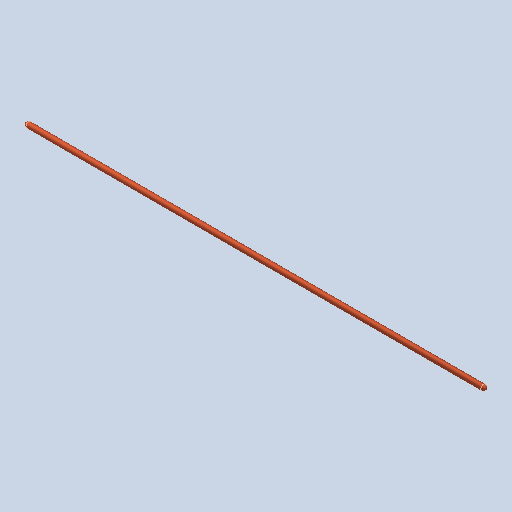
# Autodesk Inventor part: Heat Pipe 250 mm
Saved by Autodesk Inventor 2026.2 (Build 302298010, 298A)
## iProperties
Created: 2026-04-26
Part Number: Heat Pipe 250 mm
Material: Copper, Alloy
Document SubType Name: Modeling
Designer: piete
Density: 8.92 g/cm^3
Appearance: Copper - Satin
Author: piete
Autodesk Inventor part; units mm, degrees
ref_plane "YZ Plane" through (0, 0, 0) normal (1, 0, 0) x (0, 1, 0)
ref_plane "XZ Plane" through (0, 0, 0) normal (0, 1, 0) x (-1, 0, 0)
ref_plane "XY Plane" through (0, 0, 0) normal (0, 0, 1) x (1, 0, 0)
sketch "Sketch1" plane through (0, 0, 0) normal (1, 0, 0) x (0, 1, 0)
  circle A0 centre (0, 0) radius 1.5
  dimension "d0" = 3
  constraints: 1 centre point, 1 coincident
  measures "d0" diameter of A0
extrude "Extrusion1" add sketch "Sketch1" along normal blind 250
fillet "Fillet1" radius 1.5 2 edges at (250, -1.5, 0) (0, -1.5, 0)
body "Solid1"
